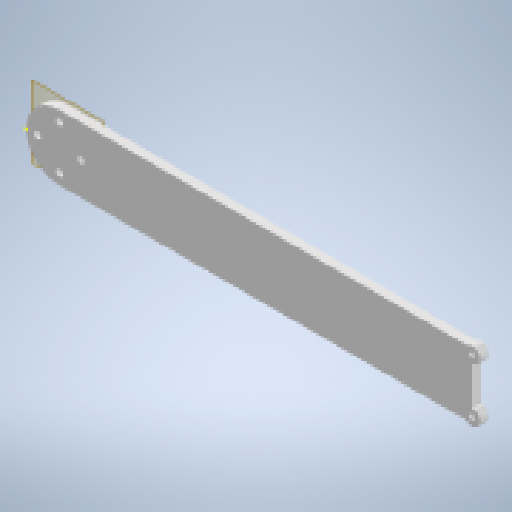
# Autodesk Inventor part: tibiaMot
Saved by Autodesk Inventor 2024 (Build 280153000, 153)
## iProperties
Created: 2024-03-17
Part Number: tibiaMot
Material: Genérico
Document SubType Name: Modeling
Designer: na_re
Density: 1 g/cm^3
Appearance: Valor por defecto
Author: na_re
Autodesk Inventor part; units mm, degrees
ref_plane "YZ Plane" through (0, 0, 0) normal (1, 0, 0) x (0, 1, 0)
ref_plane "XZ Plane" through (0, 0, 0) normal (0, 1, 0) x (-1, 0, 0)
ref_plane "XY Plane" through (0, 0, 0) normal (0, 0, 1) x (1, 0, 0)
ref_plane "Plano de trabajo1" through (0, 0, 0) normal (0, 0, 1) x (1, 0, 0)
sketch "Boceto1" plane through (0, 0, 0) normal (0, 0, 1) x (1, 0, 0)
  circle A0 centre (10.9923, 0) radius 10.9823 projected
  circle A1 centre (10.9923, 7.35) radius 1.2028 projected
  circle A2 centre (3.6423, 0) radius 1.2028 projected
  circle A3 centre (18.3423, 0) radius 1.2028 projected
  circle A4 centre (18.7153, -9.5116) radius 1.05 projected
  circle A5 centre (10.9923, -7.35) radius 1.2028 projected
  line L0 (10.9923, 0) -> (160.9923, 0)
  line L1 (10.9923, 10.9823) -> (160.9923, 10.9823)
  line L2 (10.9923, -10.9823) -> (160.9923, -10.9823)
  line L3 (160.9923, -10.9823) -> (160.9923, 10.9823)
  point P0 (0, 0)
  dimension "d0" = 150
  constraints: 8 end point, 3 horizontal, 2 point on circle, 2 tangent, 1 perpendicular
  measures "d0" distance of L0.start L0.end
extrude "Extrusión1" add sketch "Boceto1" along normal blind 3
sketch "Boceto2" plane through (0, 0, 3) normal (0, 0, 1) x (1, 0, 0)
  arc A0 (151.1597, 5.5871) -> (154.1073, 8.4343) centre (150.0864, 9.6477) ccw projected
  circle A1 centre (150.0864, -8.5523) radius 0.85 projected
  circle A2 centre (150.0864, 9.6477) radius 0.85 projected
  line L0 (160.9923, 10.9823) -> (10.9923, 10.9823) projected
  line L1 (10.9923, -10.9823) -> (160.9923, -10.9823) projected
  line L2 (160.9923, -10.9823) -> (160.9923, 10.9823) projected
  line L3 (160.9923, 10.9823) -> (10.9923, 10.9823) projected
  arc A3 (10.9923, 10.9823) -> (10.9923, -10.9823) centre (10.9923, 0) ccw projected
  circle A4 centre (18.7153, -9.5116) radius 1.05 projected
  circle A5 centre (10.9923, 7.35) radius 1.2028 projected
  circle A6 centre (3.6423, 0) radius 1.2028 projected
  circle A7 centre (10.9923, -7.35) radius 1.2028 projected
  circle A8 centre (18.3423, 0) radius 1.2028 projected
  line L4 (150.0864, 10.9823) -> (150.0864, -0.0002)
  line L5 (150.0864, -0.0002) -> (150.0864, -9.1002)
  line L6 (150.0864, -0.0002) -> (150.0864, 9.0998)
  circle A9 centre (150.0864, 9.0998) radius 0.85
  circle A10 centre (150.0864, -9.1002) radius 0.85
  circle A11 centre (150.0864, 9.0998) radius 1.8825
  circle A12 centre (150.0864, -9.1002) radius 1.8821
  point P0 (0, 0)
  point P1 (150.0864, 7.2173)
  point P2 (150.0864, -7.218)
  point P3 (150.0864, -10.9823)
  dimension "d3" = 10.9825
  dimension "d4" = 9.1
  dimension "d5" = 9.1
  dimension "d6" = 1.7
  dimension "d7" = 1.7
  constraints: 6 end point, 4 coincident, 3 centre point, 3 point on line, 1 perpendicular, 3 other
  measures "d3" distance of L4.start L4.end
  measures "d4" distance of L4.end L5.end
  measures "d5" distance of L4.end L6.end
  measures "d6" diameter of A9
  measures "d7" diameter of A10
extrude "Extrusión2" cut sketch "Boceto2" against normal blind 3 contours A10 A1 | A1 A10 | A9 L4 A2 | A2 L4 A9 | A9 L4 A2 | A2 L4 A9 | L0 L2 L1 A12 L5 L4 A11 picked at (150.2191, 8.6309) picked at (150.5614, 9.2824) picked at (149.6114, 9.2824) picked at (149.9501, 8.6317)
sketch "Boceto3" plane through (0, 0, 3) normal (0, 0, 1) x (1, 0, 0)
  point P0 (0, 0)
sketch "Boceto4" plane through (0, 0, 3) normal (0, 0, 1) x (1, 0, 0)
  circle A0 centre (18.7153, -9.5116) radius 1.05 projected
  point P0 (0, 0)
extrude "Extrusión3" add sketch "Boceto4" against normal blind 3
sketch "Boceto5" plane through (0, 0, 3) normal (0, 0, 1) x (1, 0, 0)
  circle A0 centre (150.0864, 9.0998) radius 0.85 projected
  circle A1 centre (150.0864, -9.1002) radius 0.85 projected
  circle A2 centre (150.0864, 9.0998) radius 2.6325
  circle A3 centre (150.0864, -9.1002) radius 2.632
  line L0 (150.0864, -7.218) -> (150.0864, 7.2173) projected
  circle A4 centre (18.3423, 0) radius 1.2028 projected
  circle A5 centre (10.9923, -7.35) radius 1.2028 projected
  circle A6 centre (3.6423, 0) radius 1.2028 projected
  circle A7 centre (10.9923, 7.35) radius 1.2028 projected
  arc A8 (150.0864, -10.9823) -> (150.0864, -7.218) centre (150.0864, -9.1002) ccw projected
  line L1 (150.0864, -7.218) -> (150.0864, 7.2173) projected
  arc A9 (150.0864, 7.2173) -> (150.0864, 10.9823) centre (150.0864, 9.0998) ccw projected
  line L2 (150.0864, 10.9823) -> (10.9923, 10.9823) projected
  arc A10 (10.9923, 10.9823) -> (10.9923, -10.9823) centre (10.9923, 0) ccw projected
  line L3 (10.9923, -10.9823) -> (150.0864, -10.9823) projected
  circle A11 centre (150.0864, -9.1002) radius 0.85 projected
  circle A12 centre (150.0864, 9.0998) radius 0.85 projected
  point P0 (0, 0)
  point P1 (148.2466, -10.9823)
  point P2 (150.0864, -6.4682)
  point P3 (150.0864, 6.4673)
  point P4 (148.2462, 10.9823)
  dimension "d12" = 5.265
  dimension "d13" = 5.264
  constraints: 2 centre point, 2 coincident
  measures "d12" diameter of A2
  measures "d13" diameter of A3
extrude "Extrusión4" add sketch "Boceto5" against normal blind 3 contours A2 L0 A9 L2 | A3 L3 A8 L0 picked at (149.0222, 11.1076) picked at (149.0224, -11.1076)
